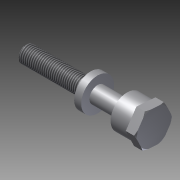
# Autodesk Inventor part: Wedge_Screw
Saved by Autodesk Inventor 2015 (Build 190159000, 159)
## iProperties
Shininess: 64.0
Angle Display Precision: 2
Document Length Units: 11272
Document Angle Units: 11279
Document Time Units: 11290
Document Mass Units: 11286
Document Length Units Precision: 3
Document Angle Units Precision: 2
Compacted: True
Created: 2004-03-19
Part Number: Wedge_Screw
Document SubType Name: Modeling
Designer: bhandley
Material: Generic
Density: 1 g/cm^3
Appearance: Default
Density: 0.0
Volumn: 0.0
Area: 0.0
PropertySet Name: Model Information
Control State: 0
Master: False
Checked Out: False
Author: bhandley
Autodesk Inventor part; units mm, degrees
ref_plane "YZ Plane" through (0, 0, 0) normal (1, 0, 0) x (0, 1, 0)
ref_plane "XZ Plane" through (0, 0, 0) normal (0, 1, 0) x (-1, 0, 0)
sketch "Sketch1" plane through (0, 0, 0) normal (0, 0, 1) x (1, 0, 0)
  line L0 (-23.9187, 7.7326) -> (57.0438, 7.7326)
  line L1 (63.3938, 7.7326) -> (63.3938, 18.8451)
  line L2 (63.3938, 18.8451) -> (72.9188, 18.8451)
  line L3 (72.9188, 18.8451) -> (72.9188, 7.7326)
  line L4 (72.9188, 7.7326) -> (112.6063, 7.7326)
  line L5 (112.6063, 7.7326) -> (112.6063, 18.8451)
  line L6 (112.6063, 18.8451) -> (149.1188, 18.8451)
  line L7 (149.1188, 18.8451) -> (149.1188, -3.3799)
  line L8 (149.1188, -3.3799) -> (-23.9187, -3.3799)
  line L9 (-23.9187, -3.3799) -> (-23.9187, 7.7326)
  line L10 (57.0438, 7.7326) -> (57.0438, 6.1451)
  line L11 (57.0438, 6.1451) -> (63.3938, 6.1451)
  line L12 (63.3938, 6.1451) -> (63.3938, 7.7326)
  dimension "d0" = 11.1125
  dimension "d1" = 22.225
  dimension "d2" = 11.1125
  dimension "d3" = 9.525
  dimension "d4" = 173.0375
  dimension "d5" = 36.5125
  dimension "d6" = 39.6875
  dimension "d7" = 6.35
  dimension "d8" = 9.525
  constraints: 26 end point, 8 parallel, 2 collinear, 1 horizontal, 1 perpendicular
  measures "d0" distance of L8.end L0.start
  measures "d1" distance of L6.end L7.end
  measures "d2" distance between parallel lines of L8 L4
  measures "d3" distance between parallel lines of L3 L1
  measures "d4" distance of L7.end L8.end
  measures "d5" distance of L5.end L6.end
  measures "d6" distance of L3.end L4.end
  measures "d7" distance of L10.end L11.end
  measures "d8" distance between parallel lines of L8 L11
revolve "Revolution1" add sketch "Sketch1" angle 360 about axis through (149.1188, -3.3799, 0) along (-1, 0, 0)
chamfer "Chamfer1" distance 1.5875 angle 45 1 edges at (-23.9187, -14.4924, 0)
sketch "Sketch2" plane through (149.1188, -3.3799, 0) normal (1, 0, 0) x (0, 0, -1)
  circle A0 centre (0, 0) radius 22.225 projected
  line L0 (14.4087, 21.2365) -> (25.5957, -1.8601)
  line L1 (25.5957, -1.8601) -> (11.187, -23.0966)
  line L2 (11.187, -23.0966) -> (-14.4087, -21.2365)
  line L3 (-14.4087, -21.2365) -> (-25.5957, 1.8601)
  line L4 (-25.5957, 1.8601) -> (-11.187, 23.0966)
  line L5 (-11.187, 23.0966) -> (14.4087, 21.2365)
  dimension "d12" = 44.45
  constraints: 12 end point, 1 coincident, 11 other
  measures "d12" distance between parallel lines of L2 L5
extrude "Extrusion1" add sketch "Sketch2" against normal blind 12.7 contours A0 L0 L1 | A0 L5 L0 | L1 L2 A0 | A0 L4 L5 | L2 L3 A0 | A0 L3 L4
ref_plane "Work Plane1" through (130.8625, -3.3799, 0) normal (0, 0, 1) x (1, 0, 0)
sketch "Sketch3" plane through (130.8625, -3.3799, 0) normal (0, 0, 1) x (1, 0, 0)
  line L0 (18.2563, 23.0966) -> (5.5563, 23.0966) projected
  line L1 (18.2563, 1.8601) -> (18.2563, 23.0966) projected
  line L2 (12.9718, 32.2495) -> (24.7507, 11.8479)
  line L3 (12.9718, 32.2495) -> (24.7507, 32.2495)
  line L4 (24.7507, 32.2495) -> (24.7507, 11.8479)
  line L5 (-172.7344, 0) -> (78.6103, 0) projected
  dimension "d16" = 30
  constraints: 6 end point, 2 perpendicular, 1 point on line
  measures "d16" angle of L2 L1
revolve "Revolution2" cut sketch "Sketch3" angle 360 about axis through (130.8625, -3.3799, 0) along (1, 0, 0)
thread "Thread1" size "7/8-9 UNC" class "1A" standard "ANSI Unified Screw Threads" full length
body "Solid1"
